Autodesk Inventor part; units mm, degrees
(part 4 of 4)
  line L479 (-28.5, 4.4019) -> (-31.5, 4.4019)
  line L480 (-23.5, 4.4019) -> (-25, 7)
  line L481 (-25, 7) -> (-23.5, 9.5981)
  line L482 (-23.5, 9.5981) -> (-20.5, 9.5981)
  line L483 (-20.5, 9.5981) -> (-19, 7)
  line L484 (-19, 7) -> (-20.5, 4.4019)
  line L485 (-20.5, 4.4019) -> (-23.5, 4.4019)
  line L486 (-39.5, 4.4019) -> (-41, 7)
  line L487 (-41, 7) -> (-39.5, 9.5981)
  line L488 (-39.5, 9.5981) -> (-36.5, 9.5981)
  line L489 (-36.5, 9.5981) -> (-35, 7)
  line L490 (-35, 7) -> (-36.5, 4.4019)
  line L491 (-36.5, 4.4019) -> (-39.5, 4.4019)
  line L492 (-55.5, 4.4019) -> (-57, 7)
  line L493 (-57, 7) -> (-55.5, 9.5981)
  line L494 (-55.5, 9.5981) -> (-52.5, 9.5981)
  line L495 (-52.5, 9.5981) -> (-51, 7)
  line L496 (-51, 7) -> (-52.5, 4.4019)
  line L497 (-52.5, 4.4019) -> (-55.5, 4.4019)
  line L498 (-71.5, 4.4019) -> (-73, 7)
  line L499 (-73, 7) -> (-71.5, 9.5981)
  line L500 (-71.5, 9.5981) -> (-68.5, 9.5981)
  line L501 (-68.5, 9.5981) -> (-67, 7)
  line L502 (-67, 7) -> (-68.5, 4.4019)
  line L503 (-68.5, 4.4019) -> (-71.5, 4.4019)
  line L504 (-11.5, 11.3301) -> (-13, 13.9282)
  line L505 (-13, 13.9282) -> (-11.5, 16.5263)
  line L506 (-11.5, 16.5263) -> (-8.5, 16.5263)
  line L507 (-8.5, 16.5263) -> (-7, 13.9282)
  line L508 (-7, 13.9282) -> (-8.5, 11.3301)
  line L509 (-8.5, 11.3301) -> (-11.5, 11.3301)
  line L510 (-27.5, 11.3301) -> (-29, 13.9282)
  line L511 (-29, 13.9282) -> (-27.5, 16.5263)
  line L512 (-27.5, 16.5263) -> (-24.5, 16.5263)
  line L513 (-24.5, 16.5263) -> (-23, 13.9282)
  line L514 (-23, 13.9282) -> (-24.5, 11.3301)
  line L515 (-24.5, 11.3301) -> (-27.5, 11.3301)
  line L516 (-43.5, 11.3301) -> (-45, 13.9282)
  line L517 (-45, 13.9282) -> (-43.5, 16.5263)
  line L518 (-43.5, 16.5263) -> (-40.5, 16.5263)
  line L519 (-40.5, 16.5263) -> (-39, 13.9282)
  line L520 (-39, 13.9282) -> (-40.5, 11.3301)
  line L521 (-40.5, 11.3301) -> (-43.5, 11.3301)
  line L522 (-59.5, 11.3301) -> (-61, 13.9282)
  line L523 (-61, 13.9282) -> (-59.5, 16.5263)
  line L524 (-59.5, 16.5263) -> (-56.5, 16.5263)
  line L525 (-56.5, 16.5263) -> (-55, 13.9282)
  line L526 (-55, 13.9282) -> (-56.5, 11.3301)
  line L527 (-56.5, 11.3301) -> (-59.5, 11.3301)
  line L528 (-75.5, 11.3301) -> (-77, 13.9282)
  line L529 (-77, 13.9282) -> (-75.5, 16.5263)
  line L530 (-75.5, 16.5263) -> (-72.5, 16.5263)
  line L531 (-72.5, 16.5263) -> (-71, 13.9282)
  line L532 (-71, 13.9282) -> (-72.5, 11.3301)
  line L533 (-72.5, 11.3301) -> (-75.5, 11.3301)
  line L534 (-15.5, 18.2583) -> (-17, 20.8564)
  line L535 (-17, 20.8564) -> (-15.5, 23.4545)
  line L536 (-15.5, 23.4545) -> (-12.5, 23.4545)
  line L537 (-12.5, 23.4545) -> (-11, 20.8564)
  line L538 (-11, 20.8564) -> (-12.5, 18.2583)
  line L539 (-12.5, 18.2583) -> (-15.5, 18.2583)
  line L540 (-31.5, 18.2583) -> (-33, 20.8564)
  line L541 (-33, 20.8564) -> (-31.5, 23.4545)
  line L542 (-31.5, 23.4545) -> (-28.5, 23.4545)
  line L543 (-28.5, 23.4545) -> (-27, 20.8564)
  line L544 (-27, 20.8564) -> (-28.5, 18.2583)
  line L545 (-28.5, 18.2583) -> (-31.5, 18.2583)
  line L546 (-47.5, 18.2583) -> (-49, 20.8564)
  line L547 (-49, 20.8564) -> (-47.5, 23.4545)
  line L548 (-47.5, 23.4545) -> (-44.5, 23.4545)
  line L549 (-44.5, 23.4545) -> (-43, 20.8564)
  line L550 (-43, 20.8564) -> (-44.5, 18.2583)
  line L551 (-44.5, 18.2583) -> (-47.5, 18.2583)
  line L552 (-63.5, 18.2583) -> (-65, 20.8564)
  line L553 (-65, 20.8564) -> (-63.5, 23.4545)
  line L554 (-63.5, 23.4545) -> (-60.5, 23.4545)
  line L555 (-60.5, 23.4545) -> (-59, 20.8564)
  line L556 (-59, 20.8564) -> (-60.5, 18.2583)
  line L557 (-60.5, 18.2583) -> (-63.5, 18.2583)
  line L558 (-79.5, 18.2583) -> (-81, 20.8564)
  line L559 (-81, 20.8564) -> (-79.5, 23.4545)
  line L560 (-79.5, 23.4545) -> (-76.5, 23.4545)
  line L561 (-76.5, 23.4545) -> (-75, 20.8564)
  line L562 (-75, 20.8564) -> (-76.5, 18.2583)
  line L563 (-76.5, 18.2583) -> (-79.5, 18.2583)
  line L564 (-80.5, 30.5263) -> (-79, 27.9282)
  line L565 (-79, 27.9282) -> (-80.5, 25.3301)
  line L566 (-80.5, 25.3301) -> (-83.5, 25.3301)
  line L567 (-83.5, 25.3301) -> (-85, 27.9282)
  line L568 (-85, 27.9282) -> (-83.5, 30.5263)
  line L569 (-83.5, 30.5263) -> (-80.5, 30.5263)
  line L570 (-51.5, 25.3301) -> (-53, 27.9282)
  line L571 (-53, 27.9282) -> (-51.5, 30.5263)
  line L572 (-51.5, 30.5263) -> (-48.5, 30.5263)
  line L573 (-48.5, 30.5263) -> (-47, 27.9282)
  line L574 (-47, 27.9282) -> (-48.5, 25.3301)
  line L575 (-48.5, 25.3301) -> (-51.5, 25.3301)
  line L576 (-67.5, 30.5263) -> (-64.5, 30.5263)
  line L577 (-64.5, 30.5263) -> (-63, 27.9282)
  line L578 (-63, 27.9282) -> (-64.5, 25.3301)
  line L579 (-64.5, 25.3301) -> (-67.5, 25.3301)
  line L580 (-67.5, 25.3301) -> (-69, 27.9282)
  line L581 (-69, 27.9282) -> (-67.5, 30.5263)
  line L582 (-35, 34.8564) -> (-36.5, 32.2583)
  line L583 (-36.5, 32.2583) -> (-39.5, 32.2583)
  line L584 (-39.5, 32.2583) -> (-41, 34.8564)
  line L585 (-41, 34.8564) -> (-39.5, 37.4545)
  line L586 (-39.5, 37.4545) -> (-36.5, 37.4545)
  line L587 (-36.5, 37.4545) -> (-35, 34.8564)
  line L588 (-55.5, 37.4545) -> (-52.5, 37.4545)
  line L589 (-52.5, 37.4545) -> (-51, 34.8564)
  line L590 (-51, 34.8564) -> (-52.5, 32.2583)
  line L591 (-52.5, 32.2583) -> (-55.5, 32.2583)
  line L592 (-55.5, 32.2583) -> (-57, 34.8564)
  line L593 (-57, 34.8564) -> (-55.5, 37.4545)
  line L594 (-71.5, 37.4545) -> (-68.5, 37.4545)
  line L595 (-68.5, 37.4545) -> (-67, 34.8564)
  line L596 (-67, 34.8564) -> (-68.5, 32.2583)
  line L597 (-68.5, 32.2583) -> (-71.5, 32.2583)
  line L598 (-71.5, 32.2583) -> (-73, 34.8564)
  line L599 (-73, 34.8564) -> (-71.5, 37.4545)
  line L600 (-15.5, 37.4545) -> (-12.5, 37.4545)
  line L601 (-12.5, 37.4545) -> (-11, 34.8564)
  line L602 (-11, 34.8564) -> (-12.5, 32.2583)
  line L603 (-12.5, 32.2583) -> (-15.5, 32.2583)
  line L604 (-15.5, 32.2583) -> (-17, 34.8564)
  line L605 (-17, 34.8564) -> (-15.5, 37.4545)
  line L606 (-35.5, 30.5263) -> (-32.5, 30.5263)
  line L607 (-32.5, 30.5263) -> (-31, 27.9282)
  line L608 (-31, 27.9282) -> (-32.5, 25.3301)
  line L609 (-32.5, 25.3301) -> (-35.5, 25.3301)
  line L610 (-35.5, 25.3301) -> (-37, 27.9282)
  line L611 (-37, 27.9282) -> (-35.5, 30.5263)
  line L612 (-20.5, 37.4545) -> (-19, 34.8564)
  line L613 (-19, 34.8564) -> (-20.5, 32.2583)
  line L614 (-20.5, 32.2583) -> (-23.5, 32.2583)
  line L615 (-23.5, 32.2583) -> (-25, 34.8564)
  line L616 (-25, 34.8564) -> (-23.5, 37.4545)
  line L617 (-23.5, 37.4545) -> (-20.5, 37.4545)
  line L618 (-11.5, 25.3301) -> (-13, 27.9282)
  line L619 (-13, 27.9282) -> (-11.5, 30.5263)
  line L620 (-11.5, 30.5263) -> (-8.5, 30.5263)
  line L621 (-8.5, 30.5263) -> (-7, 27.9282)
  line L622 (-7, 27.9282) -> (-8.5, 25.3301)
  line L623 (-8.5, 25.3301) -> (-11.5, 25.3301)
  line L624 (-80.5, 44.5263) -> (-79, 41.9282)
  line L625 (-79, 41.9282) -> (-80.5, 39.3301)
  line L626 (-80.5, 39.3301) -> (-83.5, 39.3301)
  line L627 (-83.5, 39.3301) -> (-85, 41.9282)
  line L628 (-85, 41.9282) -> (-83.5, 44.5263)
  line L629 (-83.5, 44.5263) -> (-80.5, 44.5263)
  line L630 (-51.5, 39.3301) -> (-53, 41.9282)
  line L631 (-53, 41.9282) -> (-51.5, 44.5263)
  line L632 (-51.5, 44.5263) -> (-48.5, 44.5263)
  line L633 (-48.5, 44.5263) -> (-47, 41.9282)
  line L634 (-47, 41.9282) -> (-48.5, 39.3301)
  line L635 (-48.5, 39.3301) -> (-51.5, 39.3301)
  line L636 (-67.5, 44.5263) -> (-64.5, 44.5263)
  line L637 (-64.5, 44.5263) -> (-63, 41.9282)
  line L638 (-63, 41.9282) -> (-64.5, 39.3301)
  line L639 (-64.5, 39.3301) -> (-67.5, 39.3301)
  line L640 (-67.5, 39.3301) -> (-69, 41.9282)
  line L641 (-69, 41.9282) -> (-67.5, 44.5263)
  line L642 (-35, 48.8564) -> (-36.5, 46.2583)
  line L643 (-36.5, 46.2583) -> (-39.5, 46.2583)
  line L644 (-39.5, 46.2583) -> (-41, 48.8564)
  line L645 (-41, 48.8564) -> (-39.5, 51.4545)
  line L646 (-39.5, 51.4545) -> (-36.5, 51.4545)
  line L647 (-36.5, 51.4545) -> (-35, 48.8564)
  line L648 (-55.5, 51.4545) -> (-52.5, 51.4545)
  line L649 (-52.5, 51.4545) -> (-51, 48.8564)
  line L650 (-51, 48.8564) -> (-52.5, 46.2583)
  line L651 (-52.5, 46.2583) -> (-55.5, 46.2583)
  line L652 (-55.5, 46.2583) -> (-57, 48.8564)
  line L653 (-57, 48.8564) -> (-55.5, 51.4545)
  line L654 (-71.5, 51.4545) -> (-68.5, 51.4545)
  line L655 (-68.5, 51.4545) -> (-67, 48.8564)
  line L656 (-67, 48.8564) -> (-68.5, 46.2583)
  line L657 (-68.5, 46.2583) -> (-71.5, 46.2583)
  line L658 (-71.5, 46.2583) -> (-73, 48.8564)
  line L659 (-73, 48.8564) -> (-71.5, 51.4545)
  line L660 (-15.5, 51.4545) -> (-12.5, 51.4545)
  line L661 (-12.5, 51.4545) -> (-11, 48.8564)
  line L662 (-11, 48.8564) -> (-12.5, 46.2583)
  line L663 (-12.5, 46.2583) -> (-15.5, 46.2583)
  line L664 (-15.5, 46.2583) -> (-17, 48.8564)
  line L665 (-17, 48.8564) -> (-15.5, 51.4545)
  line L666 (-35.5, 44.5263) -> (-32.5, 44.5263)
  line L667 (-32.5, 44.5263) -> (-31, 41.9282)
  line L668 (-31, 41.9282) -> (-32.5, 39.3301)
  line L669 (-32.5, 39.3301) -> (-35.5, 39.3301)
  line L670 (-35.5, 39.3301) -> (-37, 41.9282)
  line L671 (-37, 41.9282) -> (-35.5, 44.5263)
  line L672 (-20.5, 51.4545) -> (-19, 48.8564)
  line L673 (-19, 48.8564) -> (-20.5, 46.2583)
  line L674 (-20.5, 46.2583) -> (-23.5, 46.2583)
  line L675 (-23.5, 46.2583) -> (-25, 48.8564)
  line L676 (-25, 48.8564) -> (-23.5, 51.4545)
  line L677 (-23.5, 51.4545) -> (-20.5, 51.4545)
  line L678 (-11.5, 39.3301) -> (-13, 41.9282)
  line L679 (-13, 41.9282) -> (-11.5, 44.5263)
  line L680 (-11.5, 44.5263) -> (-8.5, 44.5263)
  line L681 (-8.5, 44.5263) -> (-7, 41.9282)
  line L682 (-7, 41.9282) -> (-8.5, 39.3301)
  line L683 (-8.5, 39.3301) -> (-11.5, 39.3301)
  line L684 (-80.5, 58.5263) -> (-79, 55.9282)
  line L685 (-79, 55.9282) -> (-80.5, 53.3301)
  line L686 (-80.5, 53.3301) -> (-83.5, 53.3301)
  line L687 (-83.5, 53.3301) -> (-85, 55.9282)
  line L688 (-85, 55.9282) -> (-83.5, 58.5263)
  line L689 (-83.5, 58.5263) -> (-80.5, 58.5263)
  line L690 (-51.5, 53.3301) -> (-53, 55.9282)
  line L691 (-53, 55.9282) -> (-51.5, 58.5263)
  line L692 (-51.5, 58.5263) -> (-48.5, 58.5263)
  line L693 (-48.5, 58.5263) -> (-47, 55.9282)
  line L694 (-47, 55.9282) -> (-48.5, 53.3301)
  line L695 (-48.5, 53.3301) -> (-51.5, 53.3301)
  line L696 (-67.5, 58.5263) -> (-64.5, 58.5263)
  line L697 (-64.5, 58.5263) -> (-63, 55.9282)
  line L698 (-63, 55.9282) -> (-64.5, 53.3301)
  line L699 (-64.5, 53.3301) -> (-67.5, 53.3301)
  line L700 (-67.5, 53.3301) -> (-69, 55.9282)
  line L701 (-69, 55.9282) -> (-67.5, 58.5263)
  line L702 (-35, 62.8564) -> (-36.5, 60.2583)
  line L703 (-36.5, 60.2583) -> (-39.5, 60.2583)
  line L704 (-39.5, 60.2583) -> (-41, 62.8564)
  line L705 (-41, 62.8564) -> (-39.5, 65.4545)
  line L706 (-39.5, 65.4545) -> (-36.5, 65.4545)
  line L707 (-36.5, 65.4545) -> (-35, 62.8564)
  line L708 (-55.5, 65.4545) -> (-52.5, 65.4545)
  line L709 (-52.5, 65.4545) -> (-51, 62.8564)
  line L710 (-51, 62.8564) -> (-52.5, 60.2583)
  line L711 (-52.5, 60.2583) -> (-55.5, 60.2583)
  line L712 (-55.5, 60.2583) -> (-57, 62.8564)
  line L713 (-57, 62.8564) -> (-55.5, 65.4545)
  line L714 (-71.5, 65.4545) -> (-68.5, 65.4545)
  line L715 (-68.5, 65.4545) -> (-67, 62.8564)
  line L716 (-67, 62.8564) -> (-68.5, 60.2583)
  line L717 (-68.5, 60.2583) -> (-71.5, 60.2583)
  line L718 (-71.5, 60.2583) -> (-73, 62.8564)
  line L719 (-73, 62.8564) -> (-71.5, 65.4545)
  line L720 (-15.5, 65.4545) -> (-12.5, 65.4545)
  line L721 (-12.5, 65.4545) -> (-11, 62.8564)
  line L722 (-11, 62.8564) -> (-12.5, 60.2583)
  line L723 (-12.5, 60.2583) -> (-15.5, 60.2583)
  line L724 (-15.5, 60.2583) -> (-17, 62.8564)
  line L725 (-17, 62.8564) -> (-15.5, 65.4545)
  line L726 (-35.5, 58.5263) -> (-32.5, 58.5263)
  line L727 (-32.5, 58.5263) -> (-31, 55.9282)
  line L728 (-31, 55.9282) -> (-32.5, 53.3301)
  line L729 (-32.5, 53.3301) -> (-35.5, 53.3301)
  line L730 (-35.5, 53.3301) -> (-37, 55.9282)
  line L731 (-37, 55.9282) -> (-35.5, 58.5263)
  line L732 (-20.5, 65.4545) -> (-19, 62.8564)
  line L733 (-19, 62.8564) -> (-20.5, 60.2583)
  line L734 (-20.5, 60.2583) -> (-23.5, 60.2583)
  line L735 (-23.5, 60.2583) -> (-25, 62.8564)
  line L736 (-25, 62.8564) -> (-23.5, 65.4545)
  line L737 (-23.5, 65.4545) -> (-20.5, 65.4545)
  line L738 (-11.5, 53.3301) -> (-13, 55.9282)
  line L739 (-13, 55.9282) -> (-11.5, 58.5263)
  line L740 (-11.5, 58.5263) -> (-8.5, 58.5263)
  line L741 (-8.5, 58.5263) -> (-7, 55.9282)
  line L742 (-7, 55.9282) -> (-8.5, 53.3301)
  line L743 (-8.5, 53.3301) -> (-11.5, 53.3301)
  line L744 (-80.5, 72.5263) -> (-79, 69.9282)
  line L745 (-79, 69.9282) -> (-80.5, 67.3301)
  line L746 (-80.5, 67.3301) -> (-83.5, 67.3301)
  line L747 (-83.5, 67.3301) -> (-85, 69.9282)
  line L748 (-85, 69.9282) -> (-83.5, 72.5263)
  line L749 (-83.5, 72.5263) -> (-80.5, 72.5263)
  line L750 (-51.5, 67.3301) -> (-53, 69.9282)
  line L751 (-53, 69.9282) -> (-51.5, 72.5263)
  line L752 (-51.5, 72.5263) -> (-48.5, 72.5263)
  line L753 (-48.5, 72.5263) -> (-47, 69.9282)
  line L754 (-47, 69.9282) -> (-48.5, 67.3301)
  line L755 (-48.5, 67.3301) -> (-51.5, 67.3301)
  line L756 (-67.5, 72.5263) -> (-64.5, 72.5263)
  line L757 (-64.5, 72.5263) -> (-63, 69.9282)
  line L758 (-63, 69.9282) -> (-64.5, 67.3301)
  line L759 (-64.5, 67.3301) -> (-67.5, 67.3301)
  line L760 (-67.5, 67.3301) -> (-69, 69.9282)
  line L761 (-69, 69.9282) -> (-67.5, 72.5263)
  line L762 (-35, 76.8564) -> (-36.5, 74.2583)
  line L763 (-36.5, 74.2583) -> (-39.5, 74.2583)
  line L764 (-39.5, 74.2583) -> (-41, 76.8564)
  line L765 (-41, 76.8564) -> (-39.5, 79.4545)
  line L766 (-39.5, 79.4545) -> (-36.5, 79.4545)
  line L767 (-36.5, 79.4545) -> (-35, 76.8564)
  line L768 (-55.5, 79.4545) -> (-52.5, 79.4545)
  line L769 (-52.5, 79.4545) -> (-51, 76.8564)
  line L770 (-51, 76.8564) -> (-52.5, 74.2583)
  line L771 (-52.5, 74.2583) -> (-55.5, 74.2583)
  line L772 (-55.5, 74.2583) -> (-57, 76.8564)
  line L773 (-57, 76.8564) -> (-55.5, 79.4545)
  line L774 (-71.5, 79.4545) -> (-68.5, 79.4545)
  line L775 (-68.5, 79.4545) -> (-67, 76.8564)
  line L776 (-67, 76.8564) -> (-68.5, 74.2583)
  line L777 (-68.5, 74.2583) -> (-71.5, 74.2583)
  line L778 (-71.5, 74.2583) -> (-73, 76.8564)
  line L779 (-73, 76.8564) -> (-71.5, 79.4545)
  line L780 (-15.5, 79.4545) -> (-12.5, 79.4545)
  line L781 (-12.5, 79.4545) -> (-11, 76.8564)
  line L782 (-11, 76.8564) -> (-12.5, 74.2583)
  line L783 (-12.5, 74.2583) -> (-15.5, 74.2583)
  line L784 (-15.5, 74.2583) -> (-17, 76.8564)
  line L785 (-17, 76.8564) -> (-15.5, 79.4545)
  line L786 (-35.5, 72.5263) -> (-32.5, 72.5263)
  line L787 (-32.5, 72.5263) -> (-31, 69.9282)
  line L788 (-31, 69.9282) -> (-32.5, 67.3301)
  line L789 (-32.5, 67.3301) -> (-35.5, 67.3301)
  line L790 (-35.5, 67.3301) -> (-37, 69.9282)
  line L791 (-37, 69.9282) -> (-35.5, 72.5263)
  line L792 (-20.5, 79.4545) -> (-19, 76.8564)
  line L793 (-19, 76.8564) -> (-20.5, 74.2583)
  line L794 (-20.5, 74.2583) -> (-23.5, 74.2583)
  line L795 (-23.5, 74.2583) -> (-25, 76.8564)
  line L796 (-25, 76.8564) -> (-23.5, 79.4545)
  line L797 (-23.5, 79.4545) -> (-20.5, 79.4545)
  line L798 (-11.5, 67.3301) -> (-13, 69.9282)
  line L799 (-13, 69.9282) -> (-11.5, 72.5263)
  line L800 (-11.5, 72.5263) -> (-8.5, 72.5263)
  line L801 (-8.5, 72.5263) -> (-7, 69.9282)
  line L802 (-7, 69.9282) -> (-8.5, 67.3301)
  line L803 (-8.5, 67.3301) -> (-11.5, 67.3301)
  line L804 (-80.5, 86.5263) -> (-79, 83.9282)
  line L805 (-79, 83.9282) -> (-80.5, 81.3301)
  line L806 (-80.5, 81.3301) -> (-83.5, 81.3301)
  line L807 (-83.5, 81.3301) -> (-85, 83.9282)
  line L808 (-85, 83.9282) -> (-83.5, 86.5263)
  line L809 (-83.5, 86.5263) -> (-80.5, 86.5263)
  line L810 (-51.5, 81.3301) -> (-53, 83.9282)
  line L811 (-53, 83.9282) -> (-51.5, 86.5263)
  line L812 (-51.5, 86.5263) -> (-48.5, 86.5263)
  line L813 (-48.5, 86.5263) -> (-47, 83.9282)
  line L814 (-47, 83.9282) -> (-48.5, 81.3301)
  line L815 (-48.5, 81.3301) -> (-51.5, 81.3301)
  line L816 (-67.5, 86.5263) -> (-64.5, 86.5263)
  line L817 (-64.5, 86.5263) -> (-63, 83.9282)
  line L818 (-63, 83.9282) -> (-64.5, 81.3301)
  line L819 (-64.5, 81.3301) -> (-67.5, 81.3301)
  line L820 (-67.5, 81.3301) -> (-69, 83.9282)
  line L821 (-69, 83.9282) -> (-67.5, 86.5263)
  line L822 (-35, 90.8564) -> (-36.5, 88.2583)
  line L823 (-36.5, 88.2583) -> (-39.5, 88.2583)
  line L824 (-39.5, 88.2583) -> (-41, 90.8564)
  line L825 (-41, 90.8564) -> (-39.5, 93.4545)
  line L826 (-39.5, 93.4545) -> (-36.5, 93.4545)
  line L827 (-36.5, 93.4545) -> (-35, 90.8564)
  line L828 (-55.5, 93.4545) -> (-52.5, 93.4545)
  line L829 (-52.5, 93.4545) -> (-51, 90.8564)
  line L830 (-51, 90.8564) -> (-52.5, 88.2583)
  line L831 (-52.5, 88.2583) -> (-55.5, 88.2583)
  line L832 (-55.5, 88.2583) -> (-57, 90.8564)
  line L833 (-57, 90.8564) -> (-55.5, 93.4545)
  line L834 (-71.5, 93.4545) -> (-68.5, 93.4545)
  line L835 (-68.5, 93.4545) -> (-67, 90.8564)
  line L836 (-67, 90.8564) -> (-68.5, 88.2583)
  line L837 (-68.5, 88.2583) -> (-71.5, 88.2583)
  line L838 (-71.5, 88.2583) -> (-73, 90.8564)
  line L839 (-73, 90.8564) -> (-71.5, 93.4545)
  line L840 (-27.5, 86.5263) -> (-24.5, 86.5263)
  line L841 (-24.5, 86.5263) -> (-23, 83.9282)
  line L842 (-23, 83.9282) -> (-24.5, 81.3301)
  line L843 (-24.5, 81.3301) -> (-27.5, 81.3301)
  line L844 (-27.5, 81.3301) -> (-29, 83.9282)
  line L845 (-29, 83.9282) -> (-27.5, 86.5263)
  line L846 (-15, 83.9282) -> (-16.5, 81.3301)
  line L847 (-16.5, 81.3301) -> (-19.5, 81.3301)
  line L848 (-19.5, 81.3301) -> (-21, 83.9282)
  line L849 (-21, 83.9282) -> (-19.5, 86.5263)
  line L850 (-19.5, 86.5263) -> (-16.5, 86.5263)
  line L851 (-16.5, 86.5263) -> (-15, 83.9282)
  line L852 (-80.5, 100.5263) -> (-79, 97.9282)
  line L853 (-79, 97.9282) -> (-80.5, 95.3301)
  line L854 (-80.5, 95.3301) -> (-83.5, 95.3301)
  line L855 (-83.5, 95.3301) -> (-85, 97.9282)
  line L856 (-85, 97.9282) -> (-83.5, 100.5263)
  line L857 (-83.5, 100.5263) -> (-80.5, 100.5263)
  line L858 (-51.5, 95.3301) -> (-53, 97.9282)
  line L859 (-53, 97.9282) -> (-51.5, 100.5263)
  line L860 (-51.5, 100.5263) -> (-48.5, 100.5263)
  line L861 (-48.5, 100.5263) -> (-47, 97.9282)
  line L862 (-47, 97.9282) -> (-48.5, 95.3301)
  line L863 (-48.5, 95.3301) -> (-51.5, 95.3301)
  line L864 (-67.5, 100.5263) -> (-64.5, 100.5263)
  line L865 (-64.5, 100.5263) -> (-63, 97.9282)
  line L866 (-63, 97.9282) -> (-64.5, 95.3301)
  line L867 (-64.5, 95.3301) -> (-67.5, 95.3301)
  line L868 (-67.5, 95.3301) -> (-69, 97.9282)
  line L869 (-69, 97.9282) -> (-67.5, 100.5263)
  line L870 (-35, 104.8564) -> (-36.5, 102.2583)
  line L871 (-36.5, 102.2583) -> (-39.5, 102.2583)
  line L872 (-39.5, 102.2583) -> (-41, 104.8564)
  line L873 (-41, 104.8564) -> (-39.5, 107.4545)
  line L874 (-39.5, 107.4545) -> (-36.5, 107.4545)
  line L875 (-36.5, 107.4545) -> (-35, 104.8564)
  line L876 (-55.5, 107.4545) -> (-52.5, 107.4545)
  line L877 (-52.5, 107.4545) -> (-51, 104.8564)
  line L878 (-51, 104.8564) -> (-52.5, 102.2583)
  line L879 (-52.5, 102.2583) -> (-55.5, 102.2583)
  line L880 (-55.5, 102.2583) -> (-57, 104.8564)
  line L881 (-57, 104.8564) -> (-55.5, 107.4545)
  line L882 (-71.5, 107.4545) -> (-68.5, 107.4545)
  line L883 (-68.5, 107.4545) -> (-67, 104.8564)
  line L884 (-67, 104.8564) -> (-68.5, 102.2583)
  line L885 (-68.5, 102.2583) -> (-71.5, 102.2583)
  line L886 (-71.5, 102.2583) -> (-73, 104.8564)
  line L887 (-73, 104.8564) -> (-71.5, 107.4545)
  line L888 (-35.5, 100.5263) -> (-32.5, 100.5263)
  line L889 (-32.5, 100.5263) -> (-31, 97.9282)
  line L890 (-31, 97.9282) -> (-32.5, 95.3301)
  line L891 (-32.5, 95.3301) -> (-35.5, 95.3301)
  line L892 (-35.5, 95.3301) -> (-37, 97.9282)
  line L893 (-37, 97.9282) -> (-35.5, 100.5263)
  line L894 (-75.5, 109.3301) -> (-77, 111.9282)
  line L895 (-77, 111.9282) -> (-75.5, 114.5263)
  line L896 (-75.5, 114.5263) -> (-72.5, 114.5263)
  line L897 (-72.5, 114.5263) -> (-71, 111.9282)
  line L898 (-71, 111.9282) -> (-72.5, 109.3301)
  line L899 (-72.5, 109.3301) -> (-75.5, 109.3301)
  line L900 (-59.5, 114.5263) -> (-56.5, 114.5263)
  line L901 (-56.5, 114.5263) -> (-55, 111.9282)
  line L902 (-55, 111.9282) -> (-56.5, 109.3301)
  line L903 (-56.5, 109.3301) -> (-59.5, 109.3301)
  line L904 (-59.5, 109.3301) -> (-61, 111.9282)
  line L905 (-61, 111.9282) -> (-59.5, 114.5263)
  line L906 (-75, 118.8564) -> (-76.5, 116.2583)
  line L907 (-76.5, 116.2583) -> (-79.5, 116.2583)
  line L908 (-79.5, 116.2583) -> (-81, 118.8564)
  line L909 (-81, 118.8564) -> (-79.5, 121.4545)
  line L910 (-79.5, 121.4545) -> (-76.5, 121.4545)
  line L911 (-76.5, 121.4545) -> (-75, 118.8564)
  line L912 (-47.5, 121.4545) -> (-44.5, 121.4545)
  line L913 (-44.5, 121.4545) -> (-43, 118.8564)
  line L914 (-43, 118.8564) -> (-44.5, 116.2583)
  line L915 (-44.5, 116.2583) -> (-47.5, 116.2583)
  line L916 (-47.5, 116.2583) -> (-49, 118.8564)
  line L917 (-49, 118.8564) -> (-47.5, 121.4545)
  line L918 (-63.5, 121.4545) -> (-60.5, 121.4545)
  line L919 (-60.5, 121.4545) -> (-59, 118.8564)
  line L920 (-59, 118.8564) -> (-60.5, 116.2583)
  line L921 (-60.5, 116.2583) -> (-63.5, 116.2583)
  line L922 (-63.5, 116.2583) -> (-65, 118.8564)
  line L923 (-65, 118.8564) -> (-63.5, 121.4545)
  line L924 (-43.5, 109.3301) -> (-45, 111.9282)
  line L925 (-45, 111.9282) -> (-43.5, 114.5263)
  line L926 (-43.5, 114.5263) -> (-40.5, 114.5263)
  line L927 (-40.5, 114.5263) -> (-39, 111.9282)
  line L928 (-39, 111.9282) -> (-40.5, 109.3301)
  line L929 (-40.5, 109.3301) -> (-43.5, 109.3301)
  line L930 (-80.5, 128.5263) -> (-79, 125.9282)
  line L931 (-79, 125.9282) -> (-80.5, 123.3301)
  line L932 (-80.5, 123.3301) -> (-83.5, 123.3301)
  line L933 (-83.5, 123.3301) -> (-85, 125.9282)
  line L934 (-85, 125.9282) -> (-83.5, 128.5263)
  line L935 (-83.5, 128.5263) -> (-80.5, 128.5263)
  line L936 (-51.5, 123.3301) -> (-53, 125.9282)
  line L937 (-53, 125.9282) -> (-51.5, 128.5263)
  line L938 (-51.5, 128.5263) -> (-48.5, 128.5263)
  line L939 (-48.5, 128.5263) -> (-47, 125.9282)
  line L940 (-47, 125.9282) -> (-48.5, 123.3301)
  line L941 (-48.5, 123.3301) -> (-51.5, 123.3301)
  line L942 (-67.5, 128.5263) -> (-64.5, 128.5263)
  line L943 (-64.5, 128.5263) -> (-63, 125.9282)
  line L944 (-63, 125.9282) -> (-64.5, 123.3301)
  line L945 (-64.5, 123.3301) -> (-67.5, 123.3301)
  line L946 (-67.5, 123.3301) -> (-69, 125.9282)
  line L947 (-69, 125.9282) -> (-67.5, 128.5263)
  line L948 (-35, 132.8564) -> (-36.5, 130.2583)
  line L949 (-36.5, 130.2583) -> (-39.5, 130.2583)
  line L950 (-39.5, 130.2583) -> (-41, 132.8564)
  line L951 (-41, 132.8564) -> (-39.5, 135.4545)
  line L952 (-39.5, 135.4545) -> (-36.5, 135.4545)
  line L953 (-36.5, 135.4545) -> (-35, 132.8564)
  line L954 (-55.5, 135.4545) -> (-52.5, 135.4545)
  line L955 (-52.5, 135.4545) -> (-51, 132.8564)
  line L956 (-51, 132.8564) -> (-52.5, 130.2583)
  line L957 (-52.5, 130.2583) -> (-55.5, 130.2583)
  line L958 (-55.5, 130.2583) -> (-57, 132.8564)
  line L959 (-57, 132.8564) -> (-55.5, 135.4545)
  line L960 (-71.5, 135.4545) -> (-68.5, 135.4545)
  line L961 (-68.5, 135.4545) -> (-67, 132.8564)
  line L962 (-67, 132.8564) -> (-68.5, 130.2583)
  line L963 (-68.5, 130.2583) -> (-71.5, 130.2583)
  line L964 (-71.5, 130.2583) -> (-73, 132.8564)
  line L965 (-73, 132.8564) -> (-71.5, 135.4545)
  line L966 (-35.5, 128.5263) -> (-32.5, 128.5263)
  line L967 (-32.5, 128.5263) -> (-31, 125.9282)
  line L968 (-31, 125.9282) -> (-32.5, 123.3301)
  line L969 (-32.5, 123.3301) -> (-35.5, 123.3301)
  line L970 (-35.5, 123.3301) -> (-37, 125.9282)
  line L971 (-37, 125.9282) -> (-35.5, 128.5263)
  line L972 (0, 150) -> (0, 0)
  line L973 (0, 150) -> (-86, 150)
  line L974 (-86, 0) -> (-86, 150)
  line L975 (0, 0) -> (-86, 0)
  line L976 (-86, 0) -> (-81, 0) construction
  line L977 (-81, 0) -> (-81, 5) construction
  line L978 (-81, 5) -> (-86, 5) construction
  line L979 (-86, 5) -> (-86, 0) construction
  circle A0 centre (-81, 5) radius 1.5
  line L980 (-86, 150) -> (-81, 150) construction
  line L981 (-81, 150) -> (-81, 143) construction
  line L982 (-81, 143) -> (-86, 143) construction
  line L983 (-86, 143) -> (-86, 150) construction
  circle A1 centre (-81, 143) radius 1.5
  line L984 (-81, 5) -> (-17, 5) construction
  line L985 (-81, 5) -> (-17, 5) construction
  circle A2 centre (-17, 5) radius 1.5
  point P0 (0, 75)
  dimension "d78" = 5
  dimension "d79" = 5
  dimension "d80" = 3
  dimension "d81" = 5
  dimension "d82" = 7
  dimension "d83" = 3
  dimension "d86" = 64
  dimension "d87" = 0
  dimension "d88" = 3
  constraints: 20 end point, 4 horizontal, 4 parallel, 3 centre point, 3 coincident, 2 perpendicular, 1 collinear
  measures "d78" distance of L978.end L977.end
  measures "d79" distance of L977.end L976.end
  measures "d80" diameter of A0
  measures "d81" distance of L981.end L982.end
  measures "d82" distance of L980.end L981.end
  measures "d83" diameter of A1
  measures "d86" distance of L984.start L984.end
  measures "d87" distance between parallel lines of L984 L985
  measures "d88" diameter of A2
extrude "Estrusione9" cut sketch "Schizzo10" against normal blind 10 contours A0 | A1 | A2
